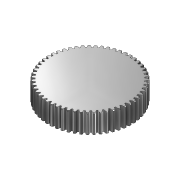
# Autodesk Inventor part: 直齿轮模板
Saved by Autodesk Inventor 2016 (Build 200138000, 138)
## iProperties
Created: 2017-07-15
Part Number: 直齿轮模板
Material: 常规
Document SubType Name: Modeling
Designer: Administrator
Density: 1 g/cm^3
Appearance: 铬 - 抛光
Author: Administrator
Autodesk Inventor part; units mm, degrees
ref_plane "YZ Plane" through (0, 0, 0) normal (1, 0, 0) x (0, 1, 0)
ref_plane "XZ Plane" through (0, 0, 0) normal (0, 1, 0) x (-1, 0, 0)
ref_plane "XY Plane" through (0, 0, 0) normal (0, 0, 1) x (1, 0, 0)
sketch "草图1" plane through (0, 0, 0) normal (0, 0, 1) x (1, 0, 0)
  circle A0 centre (0, 0) radius 52.5
  dimension "d0" = 105
  constraints: 1 centre point, 1 coincident
  measures "d0" diameter of A0
extrude "拉伸1" add sketch "草图1" along normal mid plane 26
sketch "草图2" plane through (0, 0, 13) normal (0, 0, 1) x (1, 0, 0)
  circle A0 centre (0, 0) radius 52.5 construction
  circle A1 centre (0, 0) radius 55 construction
  circle A2 centre (0, 0) radius 57 construction
  arc A3 (2.1991, 52.4539) -> (-2.1991, 52.4539) centre (0, 0) ccw
  arc A4 (0.6283, 56.9965) -> (-0.6283, 56.9965) centre (0, 0) ccw
  arc A5 (-0.6283, 56.9965) -> (-2.1991, 52.4539) centre (10.2247, 50.7008) ccw
  arc A6 (2.1991, 52.4539) -> (0.6283, 56.9965) centre (-10.2247, 50.7008) ccw
  point P0 (0, 57)
  point P1 (0, 52.5)
  point P2 (-1.5708, 54.9776)
  point P3 (1.5708, 54.9776)
  dimension "d4" = 114
  dimension "d3" = 110
  dimension "d5" = 3.1416
  dimension "d21" = 1.2566
  dimension "d22" = 4.3982
  constraints: 14 point on circle, 5 centre point, 2 coincident, 2 vertical alignment, 1 equal radius, 5 other
  measures "d3" diameter of A1
  measures "d5" distance of A1.end A1.start
  measures "d21" distance of A4.end A4.start
  measures "d22" distance of A3.end A3.start
extrude "注意：齿廓未约束" add sketch "草图2" against normal up to surface (26 mm away)
chamfer "倒角1" distance 1 angle 45 2 edges at (0, 57, 13) (0, 57, -13)
pattern_circular "环形阵列1" count 55 over 360 about axis through (0, 0, 0) along (0, 0, 1) of "注意：齿廓未约束", "倒角1"
equation "\"d0\" = 齿根圆"
equation "\"d4\" = 齿顶圆"
equation "\"d3\" = 分度圆"
equation "\"d5\" = 齿厚"
equation "\"d21\" = 0.4 * d5"
equation "\"d22\" = 1.4 * d5"
equation "\"d13\" = 齿倒角"
equation "\"齿形角\" = 20deg"
equation "\"分度圆\" = 110"
equation "\"齿顶圆\" = 114"
equation "\"齿根圆\" = 105"
equation "\"齿厚\" = 3.14159"
equation "\"齿倒角\" = 1"
